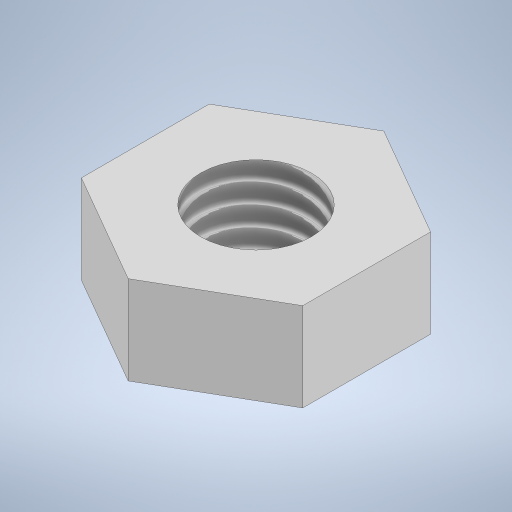
# Autodesk Inventor part: Dado esagonale
Saved by Autodesk Inventor 2023 (Build 270158000, 158)
## iProperties
Created: 2026-01-13
Part Number: Dado esagonale
Material: Generico
Document SubType Name: Modeling
Designer: Davide
Density: 1 g/cm^3
Appearance: Default
1_Materiale: − − −
2_Trattamento: − − −
3_Disegnato: D. Mitidieri
4_Controllato: C. Pirrottina
5_Approvato: S. Musella
Author: Davide
Autodesk Inventor part; units mm, degrees
ref_plane "YZ Plane" through (0, 0, 0) normal (1, 0, 0) x (0, 1, 0)
ref_plane "XZ Plane" through (0, 0, 0) normal (0, 1, 0) x (-1, 0, 0)
ref_plane "XY Plane" through (0, 0, 0) normal (0, 0, 1) x (1, 0, 0)
sketch "Schizzo1" plane through (0, 0, 0) normal (0, 1, 0) x (-1, 0, 0)
  line L0 (0, -2.8868) -> (-2.5, -1.4434)
  line L1 (-2.5, -1.4434) -> (-2.5, 1.4434)
  line L2 (-2.5, 1.4434) -> (0, 2.8868)
  line L3 (0, 2.8868) -> (2.5, 1.4434)
  line L4 (2.5, 1.4434) -> (2.5, -1.4434)
  line L5 (2.5, -1.4434) -> (0, -2.8868)
  point P0 (0, 0)
  point P1 (0, 0)
  dimension "d0" = 5
  constraints: 12 end point, 1 coincident, 1 vertical, 13 other
  measures "d0" distance between parallel lines of L1 L4
extrude "Estrusione1" add sketch "Schizzo1" along normal mid plane 2
sketch "Schizzo2" plane through (0, 1, 0) normal (0, 1, 0) x (1, 0, 0)
  circle A0 centre (0, 0) radius 1.25
  dimension "d3" = 2.5
  constraints: 1 centre point, 1 coincident
  measures "d3" diameter of A0
extrude "Estrusione2" cut sketch "Schizzo2" against normal through all
thread "Filettatura1" size "M2.5x0.45" class "6H" standard "ISO Metric profile" length 20
equation "\"d0\" = es"
equation "\"d1\" = spess"
equation "\"d3\" = d"
equation "\"es\" = 5"
equation "\"spess\" = 2"
equation "\"d\" = 2.5"
